Autodesk Fusion 360 part; units mm, degrees
note: some values were not read from the file. Chosen so that the rebuilt part matches the saved one: which face or edge a step refers to. Set by a fixed rule: which sketch regions a step uses.
(part 2 of 2)
sketch "Sketch4 (3)" plane through (0, 2.7, 0) normal (0, 1, 0) x (-1, 0, 0) in component "Finger Guides"
  line L0 (5.2, 95) -> (-5.2, 95)
  line L1 (-5.2, 95) -> (-5.2, 55)
  line L2 (-5.2, 55) -> (5.2, 55)
  line L3 (5.2, 55) -> (5.2, 95)
  line L4 (-19.8, 105) -> (-30.2, 105)
  line L5 (-30.2, 105) -> (-30.2, 55)
  line L6 (-30.2, 55) -> (-19.8, 55)
  line L7 (-19.8, 55) -> (-19.8, 105)
  line L8 (-44.8, 100) -> (-55.2, 100)
  line L9 (-55.2, 100) -> (-55.2, 55)
  line L10 (-55.2, 55) -> (-44.8, 55)
  line L11 (-44.8, 55) -> (-44.8, 100)
  line L12 (-69.8, 90) -> (-80.2, 90)
  line L13 (-80.2, 90) -> (-80.2, 55)
  line L14 (-80.2, 55) -> (-69.8, 55)
  line L15 (-69.8, 55) -> (-69.8, 90)
  line L16 (-3, 55) -> (-3, 95)
  line L17 (3, 95) -> (3, 55)
  line L18 (-22, 55) -> (-22, 105)
  line L19 (-28, 55) -> (-28, 105)
  line L20 (-47, 55) -> (-47, 100)
  line L21 (-53, 100) -> (-53, 55)
  line L22 (-72, 55) -> (-72, 90)
  line L23 (-78, 90) -> (-78, 55)
  line L24 (3, 83) -> (-3, 83)
  line L25 (-22, 93) -> (-28, 93)
  line L26 (-47, 88) -> (-53, 88)
  line L27 (-72, 78) -> (-78, 78)
  dimension "d490" = 6
  dimension "d491" = 3
  dimension "d492" = 2.2
  dimension "d493" = 6
  dimension "d494" = 6
  dimension "d495" = 6
  dimension "d496" = 2.2
  dimension "d497" = 2.2
  dimension "d498" = 2.2
  dimension "d501" = 12
  dimension "d502" = 12
  dimension "d503" = 12
  dimension "d504" = 12
  constraint vertical L16
  constraint vertical L17
  constraint coincident L0 L16.end
  constraint coincident L2 L17.end
  constraint coincident L0 L17.start
  constraint coincident L2 L16.start
  constraint coincident L6 L18.start
  constraint coincident L4 L18.end
  constraint perpendicular L4 L18
  constraint coincident L6 L19.start
  constraint coincident L4 L19.end
  constraint perpendicular L4 L19
  constraint coincident L10 L20.start
  constraint coincident L8 L20.end
  constraint perpendicular L8 L20
  constraint coincident L8 L21.start
  constraint coincident L10 L21.end
  constraint perpendicular L10 L21
  constraint coincident L12 L22.end
  constraint perpendicular L12 L22
  constraint coincident L12 L23.start
  constraint coincident L14 L23.end
  constraint perpendicular L14 L23
  constraint coincident L17 L24.start
  constraint coincident L16 L24.end
  constraint perpendicular L16 L24
  constraint coincident L18 L25.start
  constraint coincident L19 L25.end
  constraint perpendicular L19 L25
  constraint coincident L20 L26.start
  constraint coincident L21 L26.end
  constraint perpendicular L21 L26
  constraint coincident L22 L27.start
  constraint coincident L23 L27.end
  constraint perpendicular L23 L27
  measures "d490" distance of L16 L17
  measures "d491" distance of origin L17
  measures "d492" distance of L3 L17
  measures "d493" distance of L18 L19
  measures "d494" distance of L20 L21
  measures "d495" distance of L22 L23
  measures "d496" distance of L15 L22
  measures "d497" distance of L11 L20
  measures "d498" distance of L7 L18
  measures "d501" distance of L16.end L24
  measures "d502" distance of L4 L25
  measures "d503" distance of L8 L26
  measures "d504" distance of L12 L27
extrude "Extrude4'" add sketch "Sketch4 (3)" along normal blind 2.5 contours L2 L16 L17 L24 | L6 L18 L19 L25 | L10 L20 L21 L26 | L14 L22 L23 L27 bodies 7 8 13 14 in component "Finger Guides"
chamfer "Chamfer1''" distance 2.2 distance2 2.5 8 edges at (53, 2.7, 71.5) (47, 2.7, 71.5) (78, 2.7, 66.5) (72, 2.7, 66.5) (28, 2.7, 74) (22, 2.7, 74) (3, 2.7, 69) (-3, 2.7, 69) measured on face at (51, 2.7, 96) measured on face at (51, 2.7, 96) measured on face at (74, 2.7, 86) measured on face at (74, 2.7, 86) measured on face at (26, 2.7, 101) measured on face at (26, 2.7, 101) measured on face at (1, 2.7, 91) measured on face at (1, 2.7, 91) on bodies 7 8 13 14 in component "Finger Guides"
sketch "Sketch5 (3)" plane through (0, 0, 55) normal (0, 0, -1) x (-1, 0, 0) in component "Finger Guides"
  line L0 (0.3, 0.4) -> (0.3, -0.4)
  line L1 (5.2, -0.4) -> (5.2, 2.7)
  line L2 (3, 5.2) -> (-3, 5.2)
  line L3 (-5.2, 2.7) -> (-5.2, -0.4)
  line L4 (-0.3, -0.4) -> (-0.3, 0.4)
  line L5 (-0.3, 0.4) -> (0.3, 0.4)
  line L6 (4.5, 2) -> (4.5, 0.7)
  line L7 (4.5, 0.7) -> (-4.5, 0.7)
  line L8 (-4.5, 0.7) -> (-4.5, 2)
  line L9 (-4.5, 2) -> (4.5, 2)
  line L10 (1.3125, 3.2) -> (-1.3125, 3.2)
  line L11 (-1.3125, 3.2) -> (-1.3125, 4.7)
  line L12 (-1.3125, 4.7) -> (1.3125, 4.7)
  line L13 (1.3125, 4.7) -> (1.3125, 3.2)
  line L14 (-26.3125, 4.7) -> (-23.6875, 4.7)
  line L15 (-23.6875, 4.7) -> (-23.6875, 3.2)
  line L16 (-23.6875, 3.2) -> (-26.3125, 3.2)
  line L17 (-26.3125, 3.2) -> (-26.3125, 4.7)
  line L18 (-51.3125, 4.7) -> (-48.6875, 4.7)
  line L19 (-48.6875, 4.7) -> (-48.6875, 3.2)
  line L20 (-48.6875, 3.2) -> (-51.3125, 3.2)
  line L21 (-51.3125, 3.2) -> (-51.3125, 4.7)
  line L22 (-76.3125, 4.7) -> (-73.6875, 4.7)
  line L23 (-73.6875, 4.7) -> (-73.6875, 3.2)
  line L24 (-73.6875, 3.2) -> (-76.3125, 3.2)
  line L25 (-76.3125, 3.2) -> (-76.3125, 4.7)
  line L26 (-74.7, 0.4) -> (-74.7, -0.4)
  line L27 (-69.8, -0.4) -> (-69.8, 2.7)
  line L28 (-72, 5.2) -> (-78, 5.2)
  line L29 (-80.2, 2.7) -> (-80.2, -0.4)
  line L30 (-75.3, -0.4) -> (-75.3, 0.4)
  line L31 (-75.3, 0.4) -> (-74.7, 0.4)
  line L32 (-70.5, 2) -> (-70.5, 0.7)
  line L33 (-70.5, 0.7) -> (-79.5, 0.7)
  line L34 (-79.5, 0.7) -> (-79.5, 2)
  line L35 (-79.5, 2) -> (-70.5, 2)
  line L36 (-49.7, 0.4) -> (-49.7, -0.4)
  line L37 (-44.8, -0.4) -> (-44.8, 2.7)
  line L38 (-47, 5.2) -> (-53, 5.2)
  line L39 (-55.2, 2.7) -> (-55.2, -0.4)
  line L40 (-50.3, -0.4) -> (-50.3, 0.4)
  line L41 (-50.3, 0.4) -> (-49.7, 0.4)
  line L42 (-45.5, 2) -> (-45.5, 0.7)
  line L43 (-45.5, 0.7) -> (-54.5, 0.7)
  line L44 (-54.5, 0.7) -> (-54.5, 2)
  line L45 (-54.5, 2) -> (-45.5, 2)
  line L46 (-24.7, 0.4) -> (-24.7, -0.4)
  line L47 (-19.8, -0.4) -> (-19.8, 2.7)
  line L48 (-22, 5.2) -> (-28, 5.2)
  line L49 (-30.2, 2.7) -> (-30.2, -0.4)
  line L50 (-25.3, -0.4) -> (-25.3, 0.4)
  line L51 (-25.3, 0.4) -> (-24.7, 0.4)
  line L52 (-20.5, 2) -> (-20.5, 0.7)
  line L53 (-20.5, 0.7) -> (-29.5, 0.7)
  line L54 (-29.5, 0.7) -> (-29.5, 2)
  line L55 (-29.5, 2) -> (-20.5, 2)
  line L56 (5.2, -0.75) -> (5.65, -1.2)
  line L57 (5.65, -1.2) -> (8.2, -1.2)
  line L58 (8.2, -1.2) -> (8.2, -0.4)
  line L59 (8.2, -0.4) -> (5.2, -0.4)
  line L60 (-5.2, -0.4) -> (-8.2, -0.4)
  line L61 (-8.2, -0.4) -> (-8.2, -1.2)
  line L62 (-8.2, -1.2) -> (-5.65, -1.2)
  line L63 (-5.65, -1.2) -> (-5.2, -0.75)
  line L64 (-5.2, -0.75) -> (-4.75, -1.2)
  line L65 (-4.75, -1.2) -> (4.75, -1.2)
  line L66 (4.75, -1.2) -> (5.2, -0.75)
  line L67 (0.3, -0.4) -> (-0.3, -0.4)
  line L68 (-69.8, -0.75) -> (-69.35, -1.2)
  line L69 (-69.35, -1.2) -> (-66.8, -1.2)
  line L70 (-66.8, -1.2) -> (-66.8, -0.4)
  line L71 (-66.8, -0.4) -> (-69.8, -0.4)
  line L72 (-80.2, -0.4) -> (-83.2, -0.4)
  line L73 (-83.2, -0.4) -> (-83.2, -1.2)
  line L74 (-83.2, -1.2) -> (-80.65, -1.2)
  line L75 (-80.65, -1.2) -> (-80.2, -0.75)
  line L76 (-80.2, -0.75) -> (-79.75, -1.2)
  line L77 (-79.75, -1.2) -> (-70.25, -1.2)
  line L78 (-70.25, -1.2) -> (-69.8, -0.75)
  line L79 (-74.7, -0.4) -> (-75.3, -0.4)
  line L80 (-44.8, -0.75) -> (-44.35, -1.2)
  line L81 (-44.35, -1.2) -> (-41.8, -1.2)
  line L82 (-41.8, -1.2) -> (-41.8, -0.4)
  line L83 (-41.8, -0.4) -> (-44.8, -0.4)
  line L84 (-55.2, -0.4) -> (-58.2, -0.4)
  line L85 (-58.2, -0.4) -> (-58.2, -1.2)
  line L86 (-58.2, -1.2) -> (-55.65, -1.2)
  line L87 (-55.65, -1.2) -> (-55.2, -0.75)
  line L88 (-55.2, -0.75) -> (-54.75, -1.2)
  line L89 (-54.75, -1.2) -> (-45.25, -1.2)
  line L90 (-45.25, -1.2) -> (-44.8, -0.75)
  line L91 (-49.7, -0.4) -> (-50.3, -0.4)
  line L92 (-20.25, -1.2) -> (-19.8, -0.75)
  line L93 (-19.8, -0.75) -> (-19.35, -1.2)
  line L94 (-19.35, -1.2) -> (-16.8, -1.2)
  line L95 (-16.8, -1.2) -> (-16.8, -0.4)
  line L96 (-16.8, -0.4) -> (-19.8, -0.4)
  line L97 (-30.2, -0.4) -> (-33.2, -0.4)
  line L98 (-33.2, -0.4) -> (-33.2, -1.2)
  line L99 (-33.2, -1.2) -> (-30.65, -1.2)
  line L100 (-30.65, -1.2) -> (-30.2, -0.75)
  line L101 (-30.2, -0.75) -> (-29.75, -1.2)
  line L102 (-29.75, -1.2) -> (-20.25, -1.2)
  line L103 (-24.7, -0.4) -> (-25.3, -0.4)
  line L104 (5.2, 2.7) -> (3, 5.2)
  line L105 (-3, 5.2) -> (-5.2, 2.7)
  line L106 (-69.8, 2.7) -> (-72, 5.2)
  line L107 (-78, 5.2) -> (-80.2, 2.7)
  line L108 (-44.8, 2.7) -> (-47, 5.2)
  line L109 (-53, 5.2) -> (-55.2, 2.7)
  line L110 (-19.8, 2.7) -> (-22, 5.2)
  line L111 (-28, 5.2) -> (-30.2, 2.7)
  point P0 (-30.2, 2.7)
  dimension "d507" = 0.5
  dimension "d508" = 3.8875
  dimension "d509" = 2.625
  dimension "d510" = 1.5
  dimension "d511" = 2.625
  dimension "d512" = 1.5
  dimension "d513" = 0.5
  dimension "d514" = 3.8875
  dimension "d515" = 3.8875
  dimension "d516" = 0.5
  dimension "d517" = 2.625
  dimension "d518" = 1.5
  dimension "d519" = 1.5
  dimension "d520" = 2.625
  dimension "d521" = 3.8875
  dimension "d522" = 0.5
  constraint horizontal L14
  constraint vertical L15
  constraint horizontal L16
  constraint vertical L17
  constraint horizontal L18
  constraint vertical L19
  constraint horizontal L20
  constraint vertical L21
  constraint horizontal L22
  constraint vertical L23
  constraint horizontal L24
  constraint vertical L25
  measures "d507" distance of L2 L12
  measures "d508" distance of L3 L11
  measures "d509" distance of L11.end L12.end
  measures "d510" distance of L10.start L12.end
  measures "d511" distance of L22.start L22.end
  measures "d512" distance of L22.end L23.end
  measures "d513" distance of L22 L28
  measures "d514" distance of L25 L29.start
  measures "d515" distance of L21 L39.start
  measures "d516" distance of L18 L38
  measures "d517" distance of L18.start L18.end
  measures "d518" distance of L18.end L19.end
  measures "d519" distance of L14.end L15.end
  measures "d520" distance of L14.start L14.end
  measures "d521" horizontal distance of L16.end P0
  measures "d522" vertical distance of L14.start L48.end
extrude "Extrude5''" cut sketch "Sketch5 (3)" against normal up to surface (38 mm away) contours L10 L11 L12 L13 | L14 L15 L16 L17 | L18 L19 L20 L21 | L22 L23 L24 L25 bodies 13 8 7 14 in component "Finger Guides"
extrude "Extrude6'" cut 4 faces at (-1.7333, 2.7, 143.3333) (23.2667, 2.7, 157.3333) (48.2667, 2.7, 148.3333) (73.2667, 2.7, 126) along direction (0, 1, 0) up to surface end surface through (79.5, 0.7, 172) normal (0, 1, 0) offset 0 on bodies 6 10 11 15 bodies 6 10 11 15 in component "Finger Guides"
chamfer "Chamfer3" distance 2.5 distance2 7 2 edges at (1.5, -0.675, 52.25) (-1.5, -0.675, 52.25) measured on face at (-3.3792, 4.4667, 52.25) measured on face at (-3.3792, 4.4667, 52.25) on bodies 1 in component "Flex Sensor Mount"
chamfer "Chamfer4" distance 2.5 distance2 2.5 2 edges at (1.5, 0, 40.4208) (-1.5, 0, 40.4208) measured on face at (4.5389, 2.5667, 42.0324) measured on face at (4.5389, 2.5667, 42.0324) on bodies 1 in component "Flex Sensor Mount"
sketch "Sketch6 (2)" plane through (0, 2.7, 0) normal (0, 1, 0) x (-1, 0, 0) in component "Finger Guides"
  line L0 (-5.2, 83) -> (5.2, 83)
  line L1 (5.2, 83) -> (5.2, 95)
  line L2 (5.2, 95) -> (-5.2, 95)
  line L3 (-5.2, 95) -> (-5.2, 83)
  line L4 (5.2, 91) -> (-5.2, 91)
  line L5 (-30.2, 93) -> (-19.8, 93)
  line L6 (-19.8, 93) -> (-19.8, 105)
  line L7 (-19.8, 105) -> (-30.2, 105)
  line L8 (-30.2, 105) -> (-30.2, 93)
  line L9 (-55.2, 88) -> (-44.8, 88)
  line L10 (-44.8, 88) -> (-44.8, 100)
  line L11 (-44.8, 100) -> (-55.2, 100)
  line L12 (-55.2, 100) -> (-55.2, 88)
  line L13 (-80.2, 78) -> (-69.8, 78)
  line L14 (-69.8, 78) -> (-69.8, 90)
  line L15 (-69.8, 90) -> (-80.2, 90)
  line L16 (-80.2, 90) -> (-80.2, 78)
  line L17 (-19.8, 101) -> (-30.2, 101)
  line L18 (-44.8, 96) -> (-55.2, 96)
  line L19 (-69.8, 86) -> (-80.2, 86)
  dimension "d533" = 4
  dimension "d534" = 4
  dimension "d535" = 4
  dimension "d536" = 4
  constraint coincident L1 L4.start
  constraint coincident L3 L4.end
  constraint perpendicular L3 L4
  constraint coincident L6 L17.start
  constraint coincident L8 L17.end
  constraint perpendicular L8 L17
  constraint coincident L10 L18.start
  constraint coincident L12 L18.end
  constraint perpendicular L12 L18
  constraint coincident L14 L19.start
  constraint coincident L16 L19.end
  constraint perpendicular L16 L19
  measures "d533" distance of L2 L4
  measures "d534" distance of L7 L17
  measures "d535" distance of L11 L18
  measures "d536" distance of L15 L19
extrude "Extrude7'" cut sketch "Sketch6 (2)" against normal blind 1.5 contours L0 L1 L3 L4 | L5 L6 L8 L17 | L9 L10 L12 L18 | L13 L14 L16 L19 bodies 7 8 13 14 in component "Finger Guides"
component "Flex Sensor Mount" placed x (1, 0, 0) y (0, 1, 0) z (0, 0, 1) at (0, 0, 0)
component "Base" placed x (1, 0, 0) y (0, 1, 0) z (0, 0, 1) at (0, 0, 0)
component "Splay Sensor Mount" placed x (1, 0, 0) y (0, 1, 0) z (0, 0, 1) at (0, 0, 0)
component "Cam" placed x (1, 0, 0) y (0, 1, 0) z (0, 0, 1) at (0, 0, 0)
component "Finger Guides" placed x (1, 0, 0) y (0, 1, 0) z (0, 0, 1) at (0, 0, 0)
equation "d3 = ( 2.75 / 2 ) * 1 mm"
equation "d8 = d1"
equation "d9 = d1"
equation "d12 = d13 + d11"
equation "d15 = d8 / 2"
equation "d16 = d9 / 2"
equation "d18 = d17"
equation "d47 = d48 / 2"
equation "d48 = d1"
equation "d63 = -3 mm + 0.15 mm"
equation "d65 = 40 mm - 22.6 mm + 16.5 mm - 5 mm"
equation "d66 = d1 / 2 - d4"
equation "d74 = 2.75 mm - 1.125 mm"
equation "d76 = 2 mm"
equation "d78 = ( d3 + d76 - d77 ) / 2"
equation "d80 = d77"
equation "d81 = d79"
equation "d87 = d86 / 2"
equation "d119 = d133"
equation "d121 = d1 / 2"
equation "d124 = d130 / 2"
equation "d125 = d1 / 2"
equation "d127 = d216 - 0.25 mm"
equation "d128 = d124 - ( d201 + 0.125 mm )"
equation "d130 = d1 - ( 2 * ( d4 - d133 ) )"
equation "d133 = d131 / 2"
equation "d134 = d132 / 2"
equation "d200 = d126 - ( d201 + 0.125 mm )"
equation "d203 = d133 + 0.45 mm"
equation "d216 = d130 - ( 2 * ( d203 + d119 ) )"
equation "d285 = d284 / 2"
equation "d286 = d283 / 2"
equation "d288 = 0.7 mm"
equation "d289 = d296 / 2"
equation "d296 = d294 + ( d288 * 2 )"
equation "d297 = d294 / 2"
equation "d327 = d296"
equation "d329 = d327 / 2"
equation "d343 = ( d332 - d342 ) / 2"
equation "d357 = 12 mm - 5 mm"
equation "d359 = d358 / 2"
equation "d370 = d332 / 2"
equation "d372 = d371 / 2"
equation "d378 = 9 mm + ( ( 2 * 0.7 ) * 1 mm ) + ( ( 3 * 2 ) * 1 mm )"
equation "d385 = d384"
equation "d388 = d378"
equation "d394 = d384"
equation "d395 = d384"
equation "d396 = d378"
equation "d402 = d384"
equation "d403 = d384"
equation "d404 = d378"
equation "d410 = d384"
equation "d411 = d384"
equation "d414 = d378 - ( 2 * d426 )"
equation "d415 = d414"
equation "d416 = d414"
equation "d417 = d414"
equation "d427 = d426"
equation "d428 = d426"
equation "d429 = d426"
equation "d433 = d432 / 2"
equation "d434 = d431 / 2"
equation "d436 = d435"
equation "d437 = d435"
equation "d440 = d439"
equation "d441 = d438"
equation "d442 = d439"
equation "d443 = d438"
equation "d444 = d438"
equation "d445 = d439"
equation "d446 = d432"
equation "d447 = d431"
equation "d448 = d431"
equation "d449 = d432"
equation "d450 = d431"
equation "d451 = d432"
equation "d452 = d453"
equation "d453 = d435"
equation "d454 = d453"
equation "d455 = d435"
equation "d456 = d455"
equation "d457 = d455"
equation "d458 = d459"
equation "d459 = d435"
equation "d460 = d459"
equation "d461 = d466"
equation "d462 = d466"
equation "d463 = d466"
equation "d464 = d466"
equation "d465 = d466"
equation "d467 = d466"
equation "d468 = d466"
equation "d485 = d484"
equation "d486 = d484"
equation "d487 = d484"
equation "d491 = d490 / 2"
equation "d493 = d490"
equation "d494 = d490"
equation "d495 = d490"
equation "d496 = d492"
equation "d497 = d492"
equation "d498 = d492"
equation "d499 = d373 + 1 mm"
equation "d502 = d501"
equation "d503 = d502"
equation "d504 = d503"
equation "d506 = d373 + 1 mm"
equation "d511 = d509"
equation "d512 = d510"
equation "d513 = d507"
equation "d514 = d508"
equation "d515 = d508"
equation "d516 = d507"
equation "d517 = d509"
equation "d518 = d510"
equation "d519 = d510"
equation "d520 = d509"
equation "d521 = d508"
equation "d522 = d507"
equation "d534 = d533"
equation "d535 = d533"
equation "d536 = d533"
